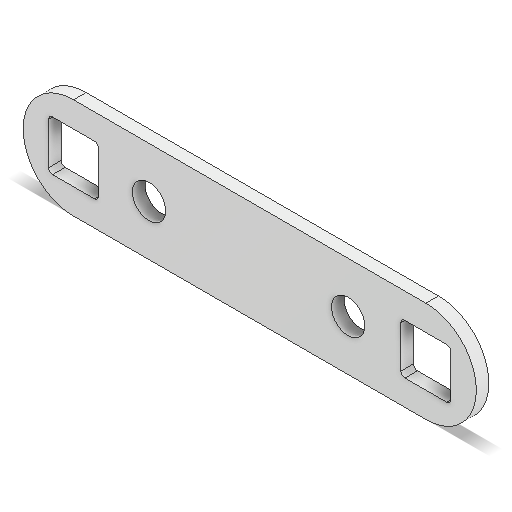
# Autodesk Inventor part: Gearbox Mirrored
Saved by Autodesk Inventor 2025.2 (Build 292293000, 293)
## iProperties
Created: 2025-02-17
Part Number: Gearbox Mirrored
Material: Acetal Resin, White
Document SubType Name: Modeling
Designer: avere
Density: 1.425 g/cm^3
Appearance: Smooth - White
Author: avere
Autodesk Inventor part; units mm, degrees
ref_plane "YZ Plane" through (0, 0, 0) normal (1, 0, 0) x (0, 1, 0)
ref_plane "XZ Plane" through (0, 0, 0) normal (0, 1, 0) x (-1, 0, 0)
ref_plane "XY Plane" through (0, 0, 0) normal (0, 0, 1) x (1, 0, 0)
sketch "Sketch1" plane through (0, 0, 0) normal (0, 0, 1) x (1, 0, 0)
  arc A0 (0, 6.35) -> (0, -6.35) centre (0, 0) ccw
  arc A1 (44.45, -6.35) -> (44.45, 6.35) centre (44.45, 0) ccw
  line L0 (0, -6.35) -> (44.45, -6.35)
  line L1 (44.45, 6.35) -> (0, 6.35)
  line L2 (-2.6416, -3.1496) -> (2.6416, -3.1496)
  line L3 (3.1496, -2.6416) -> (3.1496, 2.6416)
  line L4 (2.6416, 3.1496) -> (-2.6416, 3.1496)
  line L5 (-3.1496, 2.6416) -> (-3.1496, -2.6416)
  line L6 (-3.1496, -3.1496) -> (3.1496, 3.1496) construction
  line L7 (3.1496, -3.1496) -> (-3.1496, 3.1496) construction
  line L8 (41.8084, -3.1496) -> (47.0916, -3.1496)
  line L9 (47.5996, -2.6416) -> (47.5996, 2.6416)
  line L10 (47.0916, 3.1496) -> (41.8084, 3.1496)
  line L11 (41.3004, 2.6416) -> (41.3004, -2.6416)
  line L12 (41.3004, -3.1496) -> (47.5996, 3.1496) construction
  line L13 (47.5996, -3.1496) -> (41.3004, 3.1496) construction
  arc A2 (-2.6416, 3.1496) -> (-3.1496, 2.6416) centre (-2.6416, 2.6416) ccw
  arc A3 (3.1496, 2.6416) -> (2.6416, 3.1496) centre (2.6416, 2.6416) ccw
  arc A4 (2.6416, -3.1496) -> (3.1496, -2.6416) centre (2.6416, -2.6416) ccw
  arc A5 (-3.1496, -2.6416) -> (-2.6416, -3.1496) centre (-2.6416, -2.6416) ccw
  arc A6 (47.0916, -3.1496) -> (47.5996, -2.6416) centre (47.0916, -2.6416) ccw
  arc A7 (41.3004, -2.6416) -> (41.8084, -3.1496) centre (41.8084, -2.6416) ccw
  arc A8 (41.8084, 3.1496) -> (41.3004, 2.6416) centre (41.8084, 2.6416) ccw
  arc A9 (47.5996, 2.6416) -> (47.0916, 3.1496) centre (47.0916, 2.6416) ccw
  circle A10 centre (9.525, 0) radius 2.0955
  circle A11 centre (34.6456, 0) radius 2.0955
  dimension "d2" = 12.7
  dimension "d3" = 12.7
  dimension "d5" = 6.2992
  dimension "d6" = 6.2992
  dimension "d7" = 6.2992
  dimension "d8" = 6.2992
  dimension "d9" = 0.508
  dimension "d12" = 4.191
  dimension "d13" = 4.191
  constraints: 28 end point, 20 point on circle, 20 tangent, 16 point on line, 12 centre point, 7 equal radius, 4 midpoint, 4 parallel, 2 horizontal, 2 perpendicular, 1 horizontal alignment
  measures "d2" diameter of A0
  measures "d3" diameter of A1
  measures "d5" distance of L7.end L6.end
  measures "d6" distance of L6.end L7.start
  measures "d7" distance of L13.end L12.end
  measures "d8" distance of L12.end L13.start
  measures "d9" radius of A2
  measures "d12" diameter of A10
  measures "d13" diameter of A11
extrude "Extrusion1" add sketch "Sketch1" along normal blind 1.5875
body "Solid1"
